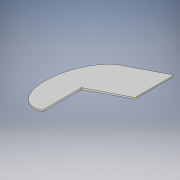
# Autodesk Inventor part: Ramp (work in progress)
Saved by Autodesk Inventor 2017 (Build 210142000, 142)
## iProperties
Created: 2018-05-09
Part Number: Ramp (work in progress)
Material: Generic
Document SubType Name: Modeling
Designer: landontracy
Density: 1 g/cm^3
Appearance: Default
Author: landontracy
Autodesk Inventor part; units mm, degrees
ref_plane "YZ Plane" through (0, 0, 0) normal (1, 0, 0) x (0, 1, 0)
ref_plane "XZ Plane" through (0, 0, 0) normal (0, 1, 0) x (-1, 0, 0)
ref_plane "XY Plane" through (0, 0, 0) normal (0, 0, 1) x (1, 0, 0)
sketch "Sketch1" plane through (0, 0, 0) normal (0, 0, 1) x (1, 0, 0)
  line L0 (-0.1602, 6.1508) -> (-481.1288, -157.3518)
  line L1 (-0.1602, -18.165) -> (-952.1117, -349.6182)
  line L2 (-481.1288, -157.3518) -> (-952.1117, -317.4598)
  line L3 (-952.1117, -317.4598) -> (-952.1117, -349.6182)
  line L4 (-0.1602, 6.1508) -> (-0.1602, -18.165)
  point P0 (0, 0)
  constraints: 10 end point, 2 vertical, 1 collinear
extrude "Extrusion1" add sketch "Sketch1" along normal blind 690.88
sketch "Sketch3" plane through (-952.1117, -317.4598, 690.88) normal (-0.3218556, 0.9467888, 0) x (0.9467888, 0.3218556, 0)
  line L0 (0, 0) -> (0, -690.88)
  arc A0 (0, 690.88) -> (0, -690.88) centre (9.8524, 0) ccw
  line L1 (1005.4529, 0) -> (0, 0) projected
  line L2 (0, 0) -> (0, 690.88)
  point P0 (1003.6249, 690.88)
  dimension "d4" = 690.88
  constraints: 4 end point, 2 point on circle, 1 centre point, 1 perpendicular, 1 vertical
  measures "d4" distance of L0.start L0.end
extrude "Extrusion2" add sketch "Sketch3" against normal blind 25.4
sketch "Sketch4" plane through (0, 0, 690.88) normal (0, 0, 1) x (1, 0, 0)
  point P0 (0, 0)
body "Solid1"
